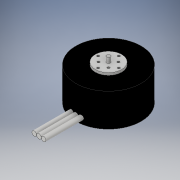
# Autodesk Inventor part: X6215S
Saved by Autodesk Inventor 2018 (Build 220112000, 112)
## iProperties
Created: 2020-02-15
Part Number: X6215S
Material: Generic
Document SubType Name: Modeling
Designer: Bunny320
Density: 1 g/cm^3
Appearance: Default
Author: Bunny320
Autodesk Inventor part; units mm, degrees
ref_plane "YZ Plane" through (0, 0, 0) normal (1, 0, 0) x (0, 1, 0)
ref_plane "XZ Plane" through (0, 0, 0) normal (0, 1, 0) x (-1, 0, 0)
ref_plane "XY Plane" through (0, 0, 0) normal (0, 0, 1) x (1, 0, 0)
sketch "Sketch1" plane through (0, 0, 0) normal (0, 0, 1) x (1, 0, 0)
  circle A0 centre (0, 0) radius 34.65
  dimension "d0" = 69.3
  constraints: 1 centre point, 1 coincident
  measures "d0" diameter of A0
extrude "Extrusion1" add sketch "Sketch1" along normal blind 35
sketch "Sketch2" plane through (0, 0, 35) normal (0, 0, 1) x (1, 0, 0)
  circle A0 centre (0, 0) radius 14
  dimension "d3" = 28
  constraints: 1 centre point, 1 coincident
  measures "d3" diameter of A0
extrude "Extrusion2" add sketch "Sketch2" along normal blind 2.5
sketch "Sketch3" plane through (0, 0, 37.5) normal (0, 0, 1) x (1, 0, 0)
  circle A0 centre (0, 0) radius 2
  dimension "d6" = 4
  constraints: 1 centre point, 1 coincident
  measures "d6" diameter of A0
extrude "Extrusion3" add sketch "Sketch3" along normal blind 5.5
sketch "Sketch4" plane through (0, 0, 0) normal (0, 1, 0) x (-1, 0, 0)
  circle A0 centre (0, 6) radius 2.5
  line L0 (-34.65, 0) -> (34.65, 0) projected
  point P0 (0, 0)
  dimension "d9" = 5
  dimension "d10" = 6
  constraints: 1 centre point
  measures "d9" diameter of A0
  measures "d10" distance from line of L0 A0.centre
extrude "Extrusion4" add sketch "Sketch4" against normal blind 74
pattern_linear "Rectangular Pattern1" count 3 spacing 5 along (1, 0, 0) of "Extrusion4" first direction both ways yes
sketch "Sketch5" plane through (0, 0, 0) normal (0, 0, 1) x (1, 0, 0)
  line L0 (10.6066, 10.6066) -> (-10.6066, 10.6066)
  line L1 (-10.6066, 10.6066) -> (-10.6066, -10.6066)
  line L2 (-10.6066, -10.6066) -> (10.6066, -10.6066)
  line L3 (10.6066, -10.6066) -> (10.6066, 10.6066)
  line L4 (10.6066, 10.6066) -> (-10.6066, -10.6066) construction
  line L5 (-10.6066, 10.6066) -> (10.6066, -10.6066) construction
  point P0 (0, 0)
  dimension "d16" = 30
  constraints: 12 end point, 4 coincident, 2 midpoint, 2 parallel, 2 perpendicular, 1 horizontal
  measures "d16" distance of L0.start L1.end
hole "Hole1" at (-10.6066, -10.6066, 0) at (-10.6066, 10.6066, 0) at (10.6066, 10.6066, 0) at (10.6066, -10.6066, 0) direction (0, 0, 1) diameter 3.242 depth 5 tip angle 118 thread size "M4x0.7" class "6H" standard "ISO Metric profile"
sketch "Sketch6" plane through (0, 0, 0) normal (0, 0, 1) x (1, 0, 0)
  circle A0 centre (0, 0) radius 5.75
  circle A1 centre (0, 0) radius 10
  dimension "d24" = 20
  dimension "d25" = 11.5
  constraints: 2 centre point, 2 coincident
  measures "d24" diameter of A1
  measures "d25" diameter of A0
extrude "Extrusion5" cut sketch "Sketch6" along normal blind 5
sketch "Sketch7" plane through (0, 0, 0) normal (0, 0, 1) x (1, 0, 0)
  line L0 (-31.5053, 13) -> (-13.3643, 6)
  line L1 (-13.3643, 6) -> (-13.3643, -6)
  line L2 (-13.3643, -6) -> (-31.5053, -13)
  line L3 (-31.5053, -13) -> (-31.5053, 13)
  point P0 (0, 0)
  dimension "d28" = 6
  dimension "d29" = 6
  dimension "d30" = 13
  constraints: 8 end point, 1 equal length, 1 parallel, 1 vertical
  measures "d28" vertical distance of point (0, 0) L1.end
  measures "d29" vertical distance of point (0, 0) L0.end
  measures "d30" vertical distance of point (0, 0) L0.start
extrude "Extrusion6" cut sketch "Sketch7" along normal blind 8
fillet "Fillet1" radius 5 4 edges at (-31.5053, -13, 4) (-13.3643, -6, 4) (-13.3643, 6, 4) (-31.5053, 13, 4)
pattern_circular "Circular Pattern1" count 4 over 360 about axis through (0, 0, -10) along (0, 0, 1) of "Extrusion6", "Fillet1"
sketch "Sketch8" plane through (0, 0, 37.5) normal (0, 0, 1) x (1, 0, 0)
  line L0 (5.3033, 5.3033) -> (0, 0) construction
  line L1 (-48.51, 0) -> (48.51, 0) projected
  point P0 (0, 11)
  dimension "d37" = 11
  dimension "d38" = 7.5
  dimension "d39" = 45
  constraints: 2 end point, 1 vertical alignment
  measures "d37" distance of L0.end point (0, 11)
  measures "d38" distance of L0.end L0.start
  measures "d39" angle of L1 L0
hole "Hole2" at (0, 11, 37.5) at (5.3033, 5.3033, 37.5) direction (0, 0, -1) diameter 2.459 depth 7.5 tip angle 118 thread size "M3x0.5" class "6H" standard "ISO Metric profile"
pattern_circular "Circular Pattern2" count 4 over 360 about axis through (0, 0, -10) along (0, 0, 1) of "Hole2"
equation "\"d29\" = d28"
body "Solid1"
